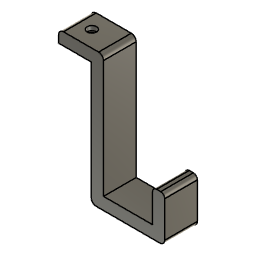
whiteboard-holder- v2 v5 (Autodesk Fusion 360 design; units mm, degrees)
Autodesk Fusion 360 part; units mm, degrees
sketch "side" plane through (0, 0, 0) normal (0, 1, 0) x (1, 0, 0)
  line L0 (0, 0) -> (27.5, 0)
  line L1 (0, 0) -> (0, 7.5)
  line L2 (0, 7.5) -> (20, 7.5)
  line L3 (20, 7.5) -> (20, 82.5)
  line L4 (34.8526, 82.5) -> (20, 82.5)
  line L5 (34.8526, 82.5) -> (65, 82.5)
  line L6 (65, 82.5) -> (65, 55)
  line L7 (65, 55) -> (57.5, 55)
  line L8 (57.5, 55) -> (57.5, 75)
  line L9 (57.5, 75) -> (27.5, 75)
  line L10 (27.5, 75) -> (27.5, 0)
  dimension "d1" = 7.5
  dimension "d2" = 7.5
  dimension "d3" = 7.5
  dimension "d4" = 20
  dimension "d5" = 7.5
  dimension "d6" = 30
  dimension "d7" = 20
  dimension "d8" = 75
  constraint coincident L0.start L1.start
  constraint horizontal L0
  constraint perpendicular L0 L1
  constraint perpendicular L1 L2
  constraint perpendicular L2 L3
  constraint perpendicular L4 L6
  constraint perpendicular L6 L7
  constraint perpendicular L7 L8
  constraint perpendicular L0 L10
  constraint perpendicular L9 L10
  measures "d1" distance of L0 L2
  measures "d2" distance of L3 L10
  measures "d3" distance of L5 L9
  measures "d4" distance of L7 L9
  measures "d5" distance of L6 L8
  measures "d6" distance of L8.end L9.end
  measures "d7" distance of L1.end L2.end
  measures "d8" distance of L0 L9
extrude "Extrude1" add sketch "side" along normal blind 20
sketch "top" plane through (0, 0, 0) normal (0, 0, 1) x (-1, 0, 0)
  line L0 (0, 0) -> (-27.5, 0)
  line L1 (-27.5, 0) -> (-27.5, -20)
  line L2 (-27.5, -20) -> (0, -20)
  line L3 (0, -20) -> (0, 0)
  line L4 (-13.75, -20) -> (-13.75, 0) construction
  circle A0 centre (-10.375, -10) radius 1.625
  circle A1 centre (-10.375, -10) radius 2.875
  line L5 (-10.375, -10) -> (0, -10) construction
  dimension "d11" = 3.25
  dimension "d12" = 5.75
  dimension "d27" = 7.5
  constraint midpoint L2 L4.start
  constraint midpoint L0 L4.end
  constraint concentric A0 A1
  constraint coincident A0.centre A1.centre
  constraint midpoint L3 L5.end
  constraint perpendicular L3 L5
  measures "d11" diameter of A0
  measures "d12" diameter of A1
  measures "d27" distance of L3 A1
fillet "Fillet1" radius 3 1 edges at (65, 10, -82.5)
fillet "Fillet2" radius 3 1 edges at (27.5, 10, 0)
fillet "Fillet3" radius 3 1 edges at (20, 10, -82.5)
fillet "Fillet4" radius 2.5 2 edges at (65, 10, -55) (57.5, 10, -55)
fillet "Fillet5" radius 3 1 edges at (0, 10, 0)
extrude "Extrude2" cut sketch "top" against normal up to surface (7.5 mm away) contours A0
extrude "Extrude3" cut sketch "top" against normal blind 2.75 contours A1
named bodies: "whiteboard-holder-v2"
